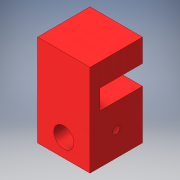
# Autodesk Inventor part: Support Overlay on Gripper Side
Saved by Autodesk Inventor 2016 (Build 200138000, 138)
## iProperties
Created: 2015-07-13
Part Number: Support Overlay on Gripper Side
Material: Aluminum 6061
Document SubType Name: Modeling
Designer: steele
Density: 2.7 g/cm^3
Appearance: Light Red
Author: steele
Autodesk Inventor part; units mm, degrees
ref_plane "YZ Plane" through (0, 0, 0) normal (1, 0, 0) x (0, 1, 0)
ref_plane "XZ Plane" through (0, 0, 0) normal (0, 1, 0) x (-1, 0, 0)
ref_plane "XY Plane" through (0, 0, 0) normal (0, 0, 1) x (1, 0, 0)
sketch "Sketch1" plane through (0, 0, 0) normal (0, 0, 1) x (1, 0, 0)
  line L0 (-25.4, -31.75) -> (25.4, -31.75)
  line L1 (25.4, -31.75) -> (25.4, 31.75)
  line L2 (25.4, 31.75) -> (-25.4, 31.75)
  line L3 (-25.4, 31.75) -> (-25.4, -31.75)
  line L4 (-25.4, -31.75) -> (25.4, 31.75) construction
  line L5 (25.4, -31.75) -> (-25.4, 31.75) construction
  point P0 (0, 0)
  dimension "Back_Height" = 63.5
  dimension "Back_Width" = 50.8
  constraints: 12 end point, 2 midpoint, 2 parallel, 1 horizontal, 1 perpendicular
  measures "Back_Height" distance of L2.end L0.start
  measures "Back_Width" distance of L1.end L2.end
extrude "Extrusion1" add sketch "Sketch1" along normal blind 50.8
sketch "Sketch2" plane through (0, 0, 0) normal (0, 0, -1) x (-1, 0, 0)
  line L0 (-25.4, -9.525) -> (25.4, -9.525)
  line L1 (25.4, -9.525) -> (25.4, 9.525)
  line L2 (25.4, 9.525) -> (-25.4, 9.525)
  line L3 (-25.4, 9.525) -> (-25.4, -9.525)
  line L4 (-25.4, -9.525) -> (25.4, 9.525) construction
  line L5 (25.4, -9.525) -> (-25.4, 9.525) construction
  point P0 (0, 0)
  dimension "Channel_Width" = 19.05
  constraints: 12 end point, 2 midpoint, 2 parallel, 1 perpendicular
  measures "Channel_Width" distance of L1.end L0.end
extrude "Extrusion2" cut sketch "Sketch2" against normal blind 41.275
sketch "Sketch3" plane through (-25.4, -31.75, 0) normal (0, -1, 0) x (1, 0, 0)
  line L0 (50.8, 41.275) -> (50.8, 0) projected
  line L1 (50.8, 50.8) -> (0, 50.8) projected
  line L2 (50.8, 0) -> (0, 0)
  line L3 (0, 0) -> (0, 50.8)
  line L4 (0, 50.8) -> (50.8, 50.8)
  line L5 (50.8, 50.8) -> (50.8, 0)
  point P0 (25.4, 0)
  constraints: 8 end point, 2 parallel, 1 horizontal, 1 perpendicular
extrude "Extrusion3" add sketch "Sketch3" along normal blind 25.4
sketch "Sketch4" plane through (0, 0, 50.8) normal (0, 0, 1) x (1, 0, 0)
  line L0 (0, 0) -> (0, -57.15) construction
  line L1 (-25.4, -57.15) -> (25.4, -57.15) construction
  line L2 (-25.4, -9.525) -> (-25.4, -57.15) construction
  line L3 (-25.4, -39.6875) -> (25.4, -39.6875) construction
  circle A0 centre (0, -39.6875) radius 9.779
  dimension "Gripper_Center_Point" = 17.4625
  dimension "d11" = 19.558
  constraints: 4 end point, 2 midpoint, 1 centre point, 1 horizontal, 1 point on line
  measures "Gripper_Center_Point" distance between parallel lines of L3 L1
  measures "d11" diameter of A0
extrude "Extrusion4" cut sketch "Sketch4" against normal through all
sketch "Sketch5" plane through (-25.4, 31.75, 0) normal (-1, 0, 0) x (0, 0, 1)
  line L0 (0, -71.4375) -> (50.8, -71.4375) construction
  line L1 (50.8, 0) -> (50.8, -88.9) construction
  line L2 (50.8, -88.9) -> (0, -88.9) construction
  line L3 (25.4, -88.9) -> (25.4, -41.275) construction
  line L4 (41.275, -41.275) -> (0, -41.275) construction
  circle A0 centre (25.4, -65.0875) radius 3.429
  point P0 (0, -31.75)
  dimension "d14" = 17.4625
  dimension "d15" = 6.858
  constraints: 4 end point, 2 midpoint, 2 point on line, 1 centre point, 1 horizontal, 1 vertical
  measures "d14" distance between parallel lines of L2 L0
  measures "d15" diameter of A0
extrude "Extrusion5" cut sketch "Sketch5" against normal through all
equation "\"d14\" = Gripper_Center_Point"
body "Solid1"
